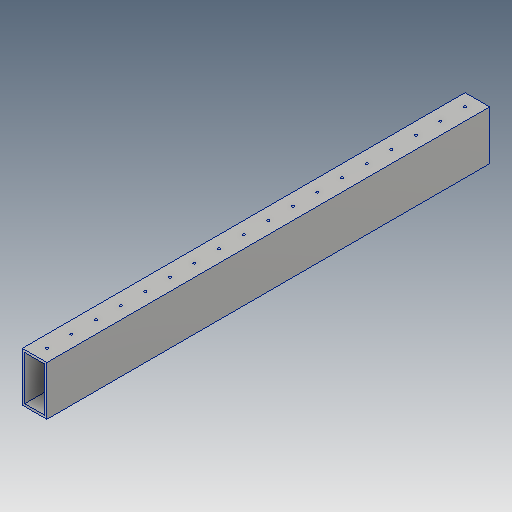
# Autodesk Inventor part: Cross Frame Rail
Saved by Autodesk Inventor 2018 (Build 220112000, 112)
## iProperties
Created: 2018-01-08
Part Number: Cross Frame Rail
Material: Aluminum 6061
Document SubType Name: Modeling
Designer: dsayers
Density: 2.7 g/cm^3
Appearance: Aluminum - Flat
Mass: 444.739 g
Surface Area: 1311.52 cm^2
Volume: 164.718 cm^3
Author: dsayers
Autodesk Inventor part; units mm, degrees
ref_plane "YZ Plane" through (0, 0, 0) normal (1, 0, 0) x (0, 1, 0)
ref_plane "XZ Plane" through (0, 0, 0) normal (0, 1, 0) x (-1, 0, 0)
ref_plane "XY Plane" through (0, 0, 0) normal (0, 0, 1) x (1, 0, 0)
sketch "Sketch1" plane through (0, 0, 0) normal (0, 0, 1) x (1, 0, 0)
  line L0 (0, 0) -> (25.4, 0)
  line L1 (25.4, 0) -> (25.4, 50.8)
  line L2 (25.4, 50.8) -> (0, 50.8)
  line L3 (0, 50.8) -> (0, 0)
  dimension "d0" = 25.4
  dimension "d1" = 50.8
  constraints: 8 end point, 2 parallel, 1 horizontal, 1 perpendicular
  measures "d0" distance of L1.end L2.end
  measures "d1" distance of L0.end L1.end
extrude "Extrusion1" add sketch "Sketch1" along normal blind 457.2
shell "Shell1" thickness 2.54 removed faces 2 at (8.4667, 33.8667, 0) at (8.4667, 33.8667, 457.2)
sketch "Sketch2" plane through (0, 50.8, 0) normal (0, 1, 0) x (1, 0, 0)
  line L0 (25.4, 0) -> (0, 0) projected
  line L1 (0, 0) -> (0, -457.2) projected
  point P0 (12.7, -12.7)
  point P1 (12.7, -38.1)
  point P2 (12.7, -63.5)
  point P3 (12.7, -88.9)
  point P4 (12.7, -114.3)
  point P5 (12.7, -139.7)
  point P6 (12.7, -165.1)
  point P7 (12.7, -190.5)
  point P8 (12.7, -215.9)
  point P9 (12.7, -241.3)
  point P10 (12.7, -266.7)
  point P11 (12.7, -292.1)
  point P12 (12.7, -317.5)
  point P13 (12.7, -342.9)
  point P14 (12.7, -368.3)
  point P15 (12.7, -393.7)
  point P16 (12.7, -419.1)
  point P17 (12.7, -444.5)
  point P18 (12.7, -469.9)
  point P19 (12.7, -495.3)
  point P20 (12.7, -520.7)
  point P21 (12.7, -546.1)
  point P22 (12.7, -571.5)
  point P23 (12.7, -596.9)
  point P24 (12.7, -622.3)
  point P25 (12.7, -647.7)
  point P26 (12.7, -673.1)
  point P27 (12.7, -698.5)
  point P28 (12.7, -723.9)
  point P29 (12.7, -749.3)
  point P30 (12.7, -774.7)
  dimension "d5" = 12.7
  dimension "d6" = 12.7
  dimension "d9" = 25.4
  constraints: 1 vertical, 30 other
  measures "d5" distance from line of L0 point (12.7, -12.7)
  measures "d6" distance from line of L1 point (12.7, -12.7)
  measures "d9" distance of point (12.7, -12.7) point (12.7, -38.1)
hole "Hole1" at (12.7, 50.8, 12.7) at (12.7, 50.8, 38.1) at (12.7, 50.8, 63.5) at (12.7, 50.8, 88.9) at (12.7, 50.8, 114.3) at (12.7, 50.8, 139.7) at (12.7, 50.8, 165.1) at (12.7, 50.8, 190.5) at (12.7, 50.8, 215.9) at (12.7, 50.8, 241.3) at (12.7, 50.8, 266.7) at (12.7, 50.8, 292.1) at (12.7, 50.8, 317.5) at (12.7, 50.8, 342.9) at (12.7, 50.8, 368.3) at (12.7, 50.8, 393.7) at (12.7, 50.8, 419.1) at (12.7, 50.8, 444.5) at (12.7, 50.8, 469.9) at (12.7, 50.8, 495.3) at (12.7, 50.8, 520.7) at (12.7, 50.8, 546.1) at (12.7, 50.8, 571.5) at (12.7, 50.8, 596.9) at (12.7, 50.8, 622.3) at (12.7, 50.8, 647.7) at (12.7, 50.8, 673.1) at (12.7, 50.8, 698.5) at (12.7, 50.8, 723.9) at (12.7, 50.8, 749.3) at (12.7, 50.8, 774.7) direction (0, -1, 0) diameter 2.54 depth 50.8 tip angle 118
body "Solid1"
